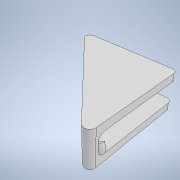
# Autodesk Inventor part: table-corners
Saved by Autodesk Inventor 2020.1 (Build 241239000, 239)
## iProperties
Created: 2019-10-01
Part Number: table-corners
Material: Generic
Document SubType Name: Modeling
Designer: Nicholas
Density: 1 g/cm^3
Appearance: Default
Author: Nicholas
Autodesk Inventor part; units mm, degrees
ref_plane "YZ Plane" through (0, 0, 0) normal (1, 0, 0) x (0, 1, 0)
ref_plane "XZ Plane" through (0, 0, 0) normal (0, 1, 0) x (-1, 0, 0)
ref_plane "XY Plane" through (0, 0, 0) normal (0, 0, 1) x (1, 0, 0)
sketch "Sketch1" plane through (0, 0, 0) normal (0, 1, 0) x (-1, 0, 0)
  line L0 (0, 0) -> (-40, 0)
  line L1 (-40, 0) -> (-40, 40)
  line L2 (-40, 40) -> (0, 0)
  dimension "d0" = 40
  dimension "d1" = 40
  dimension "d2" = 56.5685
  constraints: 6 end point, 1 horizontal, 1 vertical
  measures "d0" distance of L0.start L0.end
  measures "d1" distance of L0.end L1.end
  measures "d2" distance of L1.end L0.start
extrude "Extrusion1" add sketch "Sketch1" along normal blind 14
sketch "Sketch2" plane through (40, 0, 40) normal (-0.7071068, 0, 0.7071068) x (0.7071068, 0, 0.7071068)
  line L0 (-56.5685, 0) -> (-56.5685, 14) construction
  line L1 (-56.5685, 7) -> (0, 7) construction
  line L2 (0, 0) -> (0, 14) construction
  line L3 (-52.5685, 11) -> (-4, 11)
  line L4 (-4, 11) -> (-4, 3)
  line L5 (-4, 3) -> (-52.5685, 3)
  line L6 (-52.5685, 3) -> (-52.5685, 11)
  line L7 (-52.5685, 11) -> (-4, 3) construction
  line L8 (-4, 11) -> (-52.5685, 3) construction
  point P0 (-28.2843, 7)
  dimension "d5" = 4
  dimension "d6" = 4
  dimension "d20" = 8
  constraints: 14 end point, 5 midpoint, 2 parallel, 1 horizontal, 1 perpendicular
  measures "d5" distance between parallel lines of L2 L4
  measures "d6" distance between parallel lines of L0 L6
  measures "d20" distance between parallel lines of L5 L3
extrude "Extrusion2" cut sketch "Sketch2" against normal blind 28.75
fillet "Fillet1" radius 2 4 edges at (40, 12.5, 0) (40, 1.5, 0) (40, 7, 40) (0, 7, 0)
sketch "Sketch4" plane through (5.6569, 3, 0) normal (0.7071068, 0, 0.7071068) x (0.7071068, 0, -0.7071068)
  line L0 (-3.8204, 0) -> (-3.8204, 8) projected
  line L1 (-3.8204, 0) -> (0, 0) projected
  line L2 (0, 8) -> (0, 0) projected
  line L3 (-3.8204, 8) -> (0, 8) projected
  point P0 (-4, -3)
extrude "Extrusion3" add sketch "Sketch4" along normal blind 4
sketch "Sketch5" plane through (40, 3, 34.3431) normal (-0.7071068, 0, -0.7071068) x (-0.7071068, 0, 0.7071068)
  line L0 (3.8204, 8) -> (3.8204, 0) projected
  line L1 (3.8204, 8) -> (0, 8) projected
  line L2 (0, 0) -> (0, 8) projected
  line L3 (3.8204, 0) -> (0, 0) projected
  point P0 (4, -3)
extrude "Extrusion4" add sketch "Sketch5" along normal blind 4
sketch "Sketch6" plane through (37.2986, 3, 37.0445) normal (-0.7071068, 0, 0.7071068) x (0.7071068, 0, 0.7071068)
  line L0 (0, 8) -> (0, 0) projected
  line L1 (-4, 8) -> (0, 8) projected
  line L2 (-4, 0) -> (-4, 8) projected
  line L3 (0, 0) -> (-4, 0) projected
  point P0 (-52.5685, -3)
extrude "Extrusion5" add sketch "Sketch6" along normal up to surface (0.1796 mm away)
sketch "Sketch7" plane through (2.9555, 3, 2.7014) normal (-0.7071068, 0, 0.7071068) x (0.7071068, 0, 0.7071068)
  line L0 (0, 0) -> (0, 8) projected
  line L1 (4, 0) -> (0, 0) projected
  line L2 (4, 8) -> (4, 0) projected
  line L3 (0, 8) -> (4, 8) projected
  point P0 (-4, -3)
extrude "Extrusion6" add sketch "Sketch7" along normal up to surface (0.1796 mm away)
fillet "Fillet2" radius 2 2 edges at (37.1716, 7, 37.1716) (2.8284, 7, 2.8284)
fillet "Fillet3" radius 2 8 edges at (7.0711, 11, 4.2426) (7.0711, 3, 4.2426) (35.7574, 3, 32.9289) (35.7574, 11, 32.9289) (7.0711, 11, 1.4142) (7.0711, 3, 1.4142) (38.5858, 3, 32.9289) (38.5858, 11, 32.9289)
body "Solid1"
